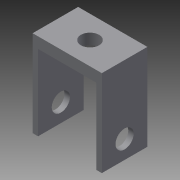
# Autodesk Inventor part: HipYaw_v2
Saved by Autodesk Inventor 2013 (Build 170138000, 138)
## iProperties
Created: 2012-11-28
Part Number: HipYaw_v2
Material: Generic
Document SubType Name: Modeling
Designer: Joe
Density: 1 g/cm^3
Author: Joe
Autodesk Inventor part; units mm, degrees
ref_plane "YZ Plane" through (0, 0, 0) normal (1, 0, 0) x (0, 1, 0)
ref_plane "XZ Plane" through (0, 0, 0) normal (0, 1, 0) x (-1, 0, 0)
ref_plane "XY Plane" through (0, 0, 0) normal (0, 0, 1) x (1, 0, 0)
sketch "Sketch1" plane through (0, 0, 0) normal (1, 0, 0) x (0, 1, 0)
  line L0 (75, 0) -> (75, -38)
  line L1 (75, -38) -> (-20, -38)
  line L2 (-20, -38) -> (-20, 0)
  line L3 (-20, 0) -> (75, 0) construction
  line L4 (75, 0) -> (75, 38)
  line L5 (75, 38) -> (-20, 38)
  line L6 (-20, 38) -> (-20, 0)
  point P0 (0, 0)
  dimension "d0" = 38
  dimension "d3" = 75
  dimension "d4" = 20
  constraints: 14 end point, 2 parallel, 2 symmetric about line, 1 perpendicular, 1 point on line, 1 vertical
  measures "d0" distance of L0.start L0.end
  measures "d3" distance from line of L0 point (0, 0)
  measures "d4" distance from line of L2 point (0, 0)
extrude "Extrusion1" add sketch "Sketch1" along normal mid plane 50
sketch "Sketch2" plane through (25, 0, 0) normal (1, 0, 0) x (0, 0, -1)
  line L0 (38, 75) -> (-38, 75) projected
  line L1 (-38, 75) -> (-38, -20) projected
  line L2 (-38, -20) -> (38, -20) projected
  line L3 (-32, -20) -> (32, -20)
  line L4 (32, -20) -> (32, 63)
  line L5 (32, 63) -> (-32, 63)
  line L6 (-32, 63) -> (-32, -20)
  line L7 (0, 63) -> (0, -20) construction
  point P0 (0, 0)
  dimension "d7" = 6
  dimension "d8" = 12
  constraints: 10 end point, 2 midpoint, 2 parallel, 2 point on line, 1 horizontal, 1 perpendicular
  measures "d7" distance between parallel lines of L1 L6
  measures "d8" distance between parallel lines of L0 L5
extrude "Extrusion2" cut sketch "Sketch2" against normal through all
sketch "Sketch3" plane through (-25, -20, 38) normal (0, 0, 1) x (1, 0, 0)
  circle A0 centre (25, 20) radius 10
  dimension "d11" = 20
  constraints: 1 centre point, 1 coincident
  measures "d11" diameter of A0
extrude "Extrusion3" cut sketch "Sketch3" against normal through all
sketch "Sketch4" plane through (-25, 75, 38) normal (0, 1, 0) x (1, 0, 0)
  circle A0 centre (25, 38) radius 10
  dimension "d15" = 20
  constraints: 1 centre point, 1 coincident
  measures "d15" diameter of A0
extrude "Extrusion4" cut sketch "Sketch4" against normal through all
move or copy body "Move Body1" bodies to move or copy 1 copy no rotation origin (0, 0, 0) rotation axis (1, 0, 0) rotation angle 90
move or copy body "Move Body2" bodies to move or copy 1 copy no rotation origin (0, 0, 0) rotation axis (0, 0, 1) rotation angle 90
body "Solid1"
